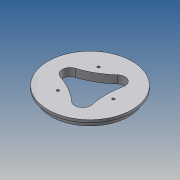
# Autodesk Inventor part: Polea Grande
Saved by Autodesk Inventor 2017 (Build 210142000, 142)
## iProperties
Part Number: Polea Grande
Material: Genérico
Document SubType Name: Modeling
Designer: FABLAB
Density: 1 g/cm^3
Appearance: Blanco
Author: FABLAB
Autodesk Inventor part; units mm, degrees
ref_plane "YZ Plane" through (0, 0, 0) normal (1, 0, 0) x (0, 1, 0)
ref_plane "XZ Plane" through (0, 0, 0) normal (0, 1, 0) x (-1, 0, 0)
ref_plane "XY Plane" through (0, 0, 0) normal (0, 0, 1) x (1, 0, 0)
sketch "Boceto1" plane through (0, 0, 0) normal (0, 0, 1) x (1, 0, 0)
  circle A0 centre (26.75, 0) radius 1.5 projected
  arc A1 (20.168, 17.783) -> (20.168, -17.783) centre (101.6471, 0) ccw projected
  arc A2 (5.3165, -26.3575) -> (20.168, -17.783) centre (11.375, -19.7021) ccw projected
  arc A3 (5.3165, -26.3575) -> (-25.4845, -8.5745) centre (-50.8235, -88.0289) ccw projected
  arc A4 (-25.4845, 8.5745) -> (-25.4845, -8.5745) centre (-22.75, 0) ccw projected
  arc A5 (-25.4845, 8.5745) -> (5.3165, 26.3575) centre (-50.8235, 88.0289) ccw projected
  arc A6 (20.168, 17.783) -> (5.3165, 26.3575) centre (11.375, 19.7021) ccw projected
  circle A7 centre (0, 0) radius 42.5 construction
  circle A8 centre (0, 0) radius 44
  circle A9 centre (-13.375, 23.1662) radius 1.5 projected
  circle A10 centre (-13.375, -23.1662) radius 1.5 projected
  point P0 (0, 0)
  dimension "d0" = 88
  constraints: 1 centre point, 1 coincident
  measures "d0" diameter of A8
extrude "Extrusión1" add sketch "Boceto1" along normal blind 6
sketch "Boceto2" plane through (0, 0, 6) normal (0, 0, 1) x (1, 0, 0)
  arc A0 (5.3165, -26.3575) -> (20.168, -17.783) centre (11.375, -19.7021) ccw projected
  arc A1 (5.3165, -26.3575) -> (-25.4845, -8.5745) centre (-50.8235, -88.0289) ccw projected
  arc A2 (-25.4845, 8.5745) -> (-25.4845, -8.5745) centre (-22.75, 0) ccw projected
  arc A3 (-25.4845, 8.5745) -> (5.3165, 26.3575) centre (-50.8235, 88.0289) ccw projected
  arc A4 (20.168, 17.783) -> (5.3165, 26.3575) centre (11.375, 19.7021) ccw projected
  arc A5 (20.168, 17.783) -> (20.168, -17.783) centre (101.6471, 0) ccw projected
  circle A6 centre (-13.375, -23.1662) radius 1.5 projected
  circle A7 centre (-13.375, 23.1662) radius 1.5 projected
  circle A8 centre (26.75, 0) radius 1.5 projected
  circle A9 centre (0, 0) radius 44 construction
  circle A10 centre (0, 0) radius 48
  point P0 (0, 0)
  dimension "d3" = 4
  constraints: 1 centre point
  measures "d3" radial gap between concentric circles of A10 A9
extrude "Extrusión2" add sketch "Boceto2" along normal blind 3 separate body
sketch "Boceto3" plane through (0, 0, 0) normal (0, 0, -1) x (-1, 0, 0)
  circle A0 centre (0, 0) radius 48 projected
  circle A1 centre (0, 0) radius 42.5
  point P0 (0, 0)
  dimension "d6" = 5.5
  constraints: 1 centre point
  measures "d6" radial gap between concentric circles of A0 A1
extrude "Extrusión3" add sketch "Boceto3" along normal blind 3 separate body
